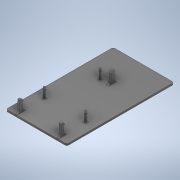
# Autodesk Inventor part: Bodemplaat
Saved by Autodesk Inventor 2022 (Build 260153000, 153)
## iProperties
Created: 2022-02-17
Part Number: Bodemplaat
Material: ABS Plastic
Document SubType Name: Modeling
Designer: woutr
Density: 1.06 g/cm^3
Appearance: Smooth - Black
Author: woutr
Autodesk Inventor part; units mm, degrees
ref_plane "YZ Plane" through (0, 0, 0) normal (1, 0, 0) x (0, 1, 0)
sketch "Sketch1" plane through (0, 0, 0) normal (0, 1, 0) x (-1, 0, 0)
  line L0 (0, 0) -> (72, 0)
  line L1 (72, 0) -> (72, -127)
  line L2 (72, -127) -> (0, -127)
  line L3 (0, -127) -> (0, 0)
  line L4 (57.1476, -114.4499) -> (13.5297, -114.4499)
  dimension "d0" = 72
  dimension "d1" = 127
  constraints: 10 end point, 2 horizontal, 2 parallel, 1 perpendicular
  measures "d0" distance of L1.end L2.end
  measures "d1" distance of L0.end L1.end
extrude "Extrusion1" add sketch "Sketch1" along normal blind 2
sketch "Sketch2" plane through (0, 2, 0) normal (0, 1, 0) x (1, 0, 0)
  circle A0 centre (-60.5, 33.8) radius 1.5
  circle A1 centre (-11.5, 33.8) radius 1.5
  circle A2 centre (-46.65, 86.2) radius 1.5
  line L0 (-71, 6) -> (-1, 6) construction
  line L1 (-1, 6) -> (-1, 88.45) construction
  line L2 (-1, 88.45) -> (-71, 88.45) construction
  line L3 (-71, 88.45) -> (-71, 6) construction
  line L4 (-72, 0) -> (0, 0) projected
  point P0 (-36, 6)
  point P1 (-36, 0)
  dimension "d34" = 3
  dimension "d83" = 70
  dimension "d84" = 82.45
  dimension "d85" = 27.8
  dimension "d86" = 10.5
  dimension "d87" = 24.35
  dimension "d88" = 10.5
  dimension "d89" = 2.25
  dimension "d90" = 6
  constraints: 8 end point, 3 centre point, 2 equal radius, 2 horizontal, 2 midpoint, 2 perpendicular, 1 horizontal alignment, 1 vertical alignment
  measures "d34" diameter of A1
  measures "d83" distance between parallel lines of L1 L3
  measures "d84" distance between parallel lines of L2 L0
  measures "d85" distance from line of L0 A1.centre
  measures "d86" distance from line of L1 A1.centre
  measures "d87" distance from line of L3 A2.centre
  measures "d88" distance from line of L3 A0.centre
  measures "d89" distance from line of L2 A2.centre
  measures "d90" distance between parallel lines of L4 L0
extrude "Extrusion8" add sketch "Sketch2" along normal blind 9
fillet "Fillet3" radius 1 3 edges at (-62, 2, -33.8) (-13, 2, -33.8) (-48.15, 2, -86.2)
sketch "Sketch8" plane through (-60.5, 11, -33.8) normal (0, 1, 0) x (1, 0, 0)
  circle A0 centre (0, 0) radius 1.25
  circle A1 centre (49, 0) radius 1.5 projected
  circle A2 centre (49, 0) radius 1.25
  circle A3 centre (13.85, 52.4) radius 1.5 projected
  circle A4 centre (13.85, 52.4) radius 1.25
  circle A5 centre (0, 0) radius 1.5 projected
  point P0 (60.5, -33.8)
  dimension "d65" = 2.5
  dimension "d66" = 2.5
  dimension "d67" = 2.5
  constraints: 3 centre point, 2 coincident, 1 concentric
  measures "d65" diameter of A0
  measures "d66" diameter of A2
  measures "d67" diameter of A4
extrude "Extrusion9" add sketch "Sketch8" along normal blind 3 contours A0 | A2 | A4
fillet "Fillet4" radius 0.5 3 edges at (-61.75, 14, -33.8) (-12.75, 14, -33.8) (-47.9, 14, -86.2)
fillet "Fillet5" radius 2 4 edges at (0, 1, 0) (-72, 1, 0) (-72, 1, -127) (0, 1, -127)
ref_plane "Work Plane1" through (-11.5, 0, -2) normal (1, 0, 0) x (0, 0, -1)
sketch "Sketch10" plane through (-11.5, 0, -2) normal (1, 0, 0) x (0, 0, -1)
  line L0 (0, 2) -> (123, 2) projected
  line L1 (-1.5, 2) -> (8.5, 2)
  arc A0 (5.7088, 3.9004) -> (8.5, 2) centre (8.5, 5) ccw
  arc A1 (-1.5, 2) -> (1.5, 5) centre (-1.5, 5) ccw
  line L2 (1.5, 5) -> (1.5, 15.9)
  line L3 (1.5, 15.9) -> (4, 15.9)
  line L4 (4, 15.9) -> (5.5, 13.9)
  line L5 (5.5, 13.9) -> (5.5, 12.9)
  line L6 (5.5, 12.9) -> (4, 12.9)
  arc A2 (4, 12.9) -> (5.7088, 3.9004) centre (28.5533, 12.9) ccw
  line L7 (-2, 2) -> (-2, 0) projected
  dimension "d92" = 10
  dimension "d96" = 1
  dimension "d98" = 3
  dimension "d100" = 2.5
  dimension "d102" = 1.5
  dimension "d103" = 3
  dimension "d117" = 10.9
  dimension "d121" = 0.5
  constraints: 12 end point, 6 point on circle, 4 tangent, 3 centre point, 3 point on line, 2 perpendicular, 1 equal radius, 1 parallel, 1 vertical, 1 vertical alignment
  measures "d92" distance of L1.start L1.end
  measures "d96" distance of L4.end L5.end
  measures "d98" radius of A0
  measures "d100" horizontal distance of L2.end L6.end
  measures "d102" distance of L5.end L6.end
  measures "d103" distance between parallel lines of L3 L6
  measures "d117" distance between parallel lines of L6 L1
  measures "d121" distance from line of L7 L1.start
extrude "Extrusion11" add sketch "Sketch10" along normal mid plane 2.5
ref_plane "Work Plane2" through (-36, 0, -2) normal (1, 0, 0) x (0, 0, -1)
mirror "Mirror1" about plane through (-36, 0, -2) normal (1, 0, 0) of "Extrusion11"
sketch "Sketch11" plane through (-36, 0, -2) normal (1, 0, 0) x (0, 0, -1)
  line L0 (0, 2) -> (123, 2) projected
  line L1 (81.95, 2) -> (91.95, 2)
  arc A0 (88.95, 5) -> (91.95, 2) centre (91.95, 5) ccw
  line L2 (88.95, 5) -> (88.95, 15.9)
  line L3 (88.95, 15.9) -> (86.45, 15.9)
  line L4 (86.45, 15.9) -> (84.95, 13.9)
  line L5 (84.95, 13.9) -> (84.95, 12.9)
  line L6 (84.95, 12.9) -> (86.45, 12.9)
  arc A1 (81.95, 2) -> (84.7412, 3.9004) centre (81.95, 5) ccw
  arc A2 (84.7412, 3.9004) -> (86.45, 12.9) centre (61.8967, 12.9) ccw
  line L7 (-2, 2) -> (-2, 0) projected
  point P0 (4, 12.9)
  dimension "d107" = 10
  dimension "d109" = 2.5
  dimension "d112" = 3
  dimension "d113" = 3
  dimension "d118" = 1
  dimension "d119" = 1.5
  dimension "d120" = 10.9
  dimension "d122" = 82.45
  constraints: 12 end point, 6 point on circle, 4 tangent, 3 centre point, 3 point on line, 2 perpendicular, 1 equal radius, 1 parallel, 1 vertical, 1 vertical alignment
  measures "d107" distance of L1.start L1.end
  measures "d109" distance of L2.end L3.end
  measures "d112" radius of A0
  measures "d113" distance between parallel lines of L3 L6
  measures "d118" distance of L4.end L5.end
  measures "d119" distance of L5.end L6.end
  measures "d120" distance between parallel lines of L1 L6
  measures "d122" distance of L6.end point (4, 12.9)
extrude "Extrusion12" add sketch "Sketch11" along normal mid plane 2.5
body "Solid1"
